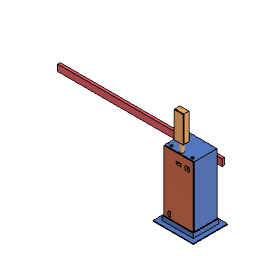
barrier (Autodesk Fusion 360 design; units mm, degrees)
part number: 2026-01-20-15-57-13-019
part number: 2026-01-20-15-58-03-444
part number: 2026-01-20-18-25-53-165
part number: 2026-01-21-16-47-12-671
part number: 2026-01-23-16-32-55-058
Autodesk Fusion 360 part; units mm, degrees
note: some values were not read from the file. Set by a fixed rule: which face or edge a step refers to.
sketch "base" plane through (0, 0, 0) normal (0, 1, 0) x (1, 0, 0) in component "base"
  line L0 (22.5, 0) -> (-22.5, 0)
  line L1 (-22.5, 0) -> (-22.5, -100)
  line L2 (-22.5, -100) -> (22.5, -100)
  line L3 (22.5, -100) -> (22.5, 0)
  line L4 (22.5, 0) -> (-22.5, -100) construction
  line L5 (-22.5, 0) -> (22.5, -100) construction
  point P0 (0, -50)
  dimension "d5" = 45
  dimension "d6" = 100
  constraint horizontal L0
  constraint perpendicular L0 L1
  constraint parallel L0 L2
  constraint parallel L1 L3
  constraint coincident L4 P0
  constraint coincident L5 P0
  constraint midpoint origin L0
  measures "d5" distance of L1.end L2.end
  measures "d6" distance of L0.end L1.end
extrude "Extrude1" add sketch "base" along normal blind 35 makes body 1 in component "base"
shell "Shell1" thickness 1.2 removed faces 1 at (-7.5, 0, 66.6667) on bodies 1 in component "base"
sketch "motor-mount" plane through (0, 33.8, 0) normal (0, -1, 0) x (1, 0, 0) in component "base"
  line L0 (21.3, 1.2) -> (21.3, 98.8)
  line L1 (21.3, 98.8) -> (-21.3, 98.8)
  line L2 (-21.3, 98.8) -> (-21.3, 1.2)
  line L3 (-21.3, 1.2) -> (21.3, 1.2)
  circle A0 centre (0, 85) radius 5
  line L4 (-22.5, 100) -> (22.5, 100)
  line L5 (0, 0) -> (0, 100) construction
  circle A1 centre (17.5, 77) radius 2
  circle A2 centre (-17.5, 77) radius 2
  circle A3 centre (13.2, 45) radius 1
  circle A4 centre (13.2, 15) radius 1
  circle A5 centre (-13.2, 45) radius 1
  circle A6 centre (-13.2, 15) radius 1
  dimension "d15" = 10
  dimension "d16" = 15
  dimension "d17" = 4
  dimension "d18" = 17.5
  dimension "d19" = 8
  dimension "d27" = 2
  dimension "d28" = 13.2
  dimension "d29" = 55
  dimension "d30" = 2
  dimension "d31" = 13.2
  dimension "d32" = 30
  constraint vertical L5.start A0.centre
  constraint coincident L5.start origin
  constraint midpoint L4 L5.end
  constraint symmetric L5 A1 A2
  constraint symmetric L5 A3 A5
  constraint symmetric L5 A4 A6
  measures "d15" diameter of A0
  measures "d16" distance of A0.centre L4
  measures "d17" diameter of A1
  measures "d18" distance of L5 A1.centre
  measures "d19" vertical distance of A0.centre A1.centre
  measures "d27" diameter of A3
  measures "d28" distance of L5 A3.centre
  measures "d29" distance of L4 A3.centre
  measures "d30" diameter of A4
  measures "d31" distance of L5 A4.centre
  measures "d32" distance of A3.centre A4.centre
extrude "Extrude2" cut sketch "motor-mount" against normal through all contours A0 bodies 1 in component "base"
extrude "Extrude3" add sketch "motor-mount" along normal blind 3 contours A1 | A2 bodies 1 in component "base"
extrude "Extrude4" add sketch "motor-mount" along normal blind 4 contours A3 | A4 | A5 | A6 bodies 1 in component "base"
sketch "Sketch1" plane through (0, 35, 0) normal (0, 1, 0) x (-1, 0, 0) in component "arm"
  circle A0 centre (0, 85) radius 5
  line L0 (-22.5, 100) -> (-22.5, 0)
  line L1 (-22.5, 0) -> (22.5, 0)
  line L2 (22.5, 0) -> (22.5, 100)
  line L3 (22.5, 100) -> (-22.5, 100)
  circle A1 centre (0, 85) radius 2.5
  line L4 (2.5, 86.6) -> (-2.5, 86.6)
  line L5 (-2.5, 86.6) -> (-2.5, 83.4)
  line L6 (-2.5, 83.4) -> (2.5, 83.4)
  line L7 (2.5, 83.4) -> (2.5, 86.6)
  line L8 (2.5, 86.6) -> (-2.5, 83.4) construction
  line L9 (-2.5, 86.6) -> (2.5, 83.4) construction
  line L10 (220, 80) -> (-30, 80)
  line L11 (-30, 80) -> (-30, 90)
  line L12 (-30, 90) -> (220, 90)
  line L13 (220, 90) -> (220, 80)
  line L14 (220, 80) -> (-30, 90) construction
  line L15 (-30, 80) -> (220, 90) construction
  point P0 (0, 85)
  point P1 (95, 85)
  dimension "d37" = 5
  dimension "d38" = 15
  dimension "d39" = 5
  dimension "d40" = 3.2
  dimension "d44" = 250
  dimension "d45" = 10
  dimension "d46" = 15
  dimension "d47" = 30
  constraint vertical origin A0.centre
  constraint horizontal L4
  constraint perpendicular L4 L5
  constraint parallel L4 L6
  constraint parallel L5 L7
  constraint coincident L8 P0
  constraint coincident L9 P0
  constraint coincident P0 A0.centre
  constraint horizontal L10
  constraint perpendicular L10 L11
  constraint parallel L10 L12
  constraint parallel L11 L13
  constraint coincident L14 P1
  constraint coincident L15 P1
  measures "d37" diameter of A1
  measures "d38" distance of L3 P0
  measures "d39" distance of L5.end L6.end
  measures "d40" distance of L4.end L5.end
  measures "d44" distance of L11.end L12.end
  measures "d45" distance of L10.end L11.end
  measures "d46" distance of L3 P1
  measures "d47" distance of P0 L11
extrude "Extrude1'" add sketch "Sketch1" along normal blind 4 separate body contours A0 | A0 L2 L10 L12 | A0 L0 L10 L12 | L0 L10 L11 L12 | L2 L10 L12 L13 | A1 L6 L7 | A1 L4 L7 | A1 L4 | A1 L6 | A1 L4 L5 | A1 L5 L6 makes body 2 in component "arm"
sketch "light-box" plane through (0, 0, 0) normal (0, 1, 0) x (1, 0, 0) in component "light-box"
  line L0 (7, -115) -> (-7, -115)
  line L1 (-7, -115) -> (-7, -155)
  line L2 (-7, -155) -> (7, -155)
  line L3 (7, -155) -> (7, -115)
  line L4 (7, -115) -> (-7, -155) construction
  line L5 (-7, -115) -> (7, -155) construction
  line L6 (-22.5, -100) -> (22.5, -100)
  circle A0 centre (0, -148) radius 4.5
  line L7 (7, -139.5) -> (-7, -139.5) construction
  circle A1 centre (0, -131) radius 4.5
  line L8 (7, -138.5) -> (-7, -138.5)
  line L9 (-7, -138.5) -> (-7, -140.5)
  line L10 (-7, -140.5) -> (7, -140.5)
  line L11 (7, -140.5) -> (7, -138.5)
  line L12 (7, -138.5) -> (-7, -140.5) construction
  line L13 (-7, -138.5) -> (7, -140.5) construction
  circle A2 centre (0, -148) radius 5.5
  circle A3 centre (0, -131) radius 5.5
  line L14 (5.7, -116.3) -> (-5.7, -116.3)
  line L15 (-5.7, -116.3) -> (-5.7, -153.7)
  line L16 (-5.7, -153.7) -> (5.7, -153.7)
  line L17 (5.7, -153.7) -> (5.7, -116.3)
  point P0 (0, -135)
  point P1 (0, -85)
  point P2 (0, -139.5)
  dimension "d55" = 14
  dimension "d56" = 40
  dimension "d57" = 15
  dimension "d61" = 9
  dimension "d65" = 7
  dimension "d66" = 8.5
  dimension "d75" = 14
  dimension "d76" = 2
  dimension "d77" = 8.5
  dimension "d78" = 1
  dimension "d79" = 1
  dimension "d146" = -1.3
  constraint horizontal L0
  constraint perpendicular L0 L1
  constraint parallel L0 L2
  constraint parallel L1 L3
  constraint coincident L4 P0
  constraint coincident L5 P0
  constraint vertical origin P0
  constraint vertical A0.centre origin
  constraint coincident L3 L7.start
  constraint coincident L1 L7.end
  constraint perpendicular L1 L7
  constraint symmetric A0 L7 A1
  constraint horizontal L8
  constraint perpendicular L8 L9
  constraint parallel L8 L10
  constraint parallel L9 L11
  constraint coincident L12 P2
  constraint coincident L13 P2
  constraint vertical origin P2
  measures "d55" distance of L1.end L2.end
  measures "d56" distance of L0.end L1.end
  measures "d57" distance of L0 L6
  measures "d61" diameter of A0
  measures "d65" distance of L2 A0.centre
  measures "d66" distance of A0.centre L7
  measures "d75" distance of L9.end L10.end
  measures "d76" distance of L8.end L9.end
  measures "d77" distance of A0.centre P2
extrude "Extrude1''" add sketch "light-box" along normal blind 8 separate body contours L0 L1 L3 L8 L14 L15 L17 | L3 L8 L10 L11 L17 | L1 L8 L9 L10 L15 | L1 L2 L3 L10 L15 L16 L17 | L8 L10 L15 L17 | L8 L14 L15 L17 | L10 L15 L16 L17 | A0 | A1 | A2 | A3 makes body 3 in component "light-box"
shell "Shell1'" thickness 1.2 removed faces 1 at (-2.3333, 0, 122.8333) on bodies 3 in component "light-box"
extrude "Extrude2'" cut sketch "light-box" along normal through all contours A0 | A1 bodies 3 in component "light-box"
sketch "pole" plane through (0, 0, 116.2) normal (0, 0, 1) x (-1, 0, 0) in component "light-box"
  line L0 (5.8, 0) -> (-5.8, 0)
  line L1 (-5.8, 0) -> (-5.8, -6.8)
  line L2 (-5.8, -6.8) -> (5.8, -6.8)
  line L3 (5.8, -6.8) -> (5.8, 0)
  circle A0 centre (0, -4) radius 2
  circle A1 centre (0, -4) radius 2.8
  dimension "d68" = 4
  dimension "d69" = 4
  dimension "d74" = 0.8
  constraint vertical origin A0.centre
  measures "d68" diameter of A0
  measures "d69" distance of origin A0.centre
extrude "Extrude3'" cut sketch "pole" against normal up to surface (1.2 mm away) contours A0 bodies 3 in component "light-box"
extrude "Extrude5" add sketch "light-box" against normal blind 4 from surface at 6.8 contours L3 L8 L10 L11 L17 | L1 L8 L9 L10 L15 | L8 L10 L15 L17 | A2 | A3 bodies 3 in component "light-box"
extrude "Extrude6" add sketch "pole" against normal up to surface (16.2 mm away) separate body contours A1 makes body 4 in component "light-box"
sketch "pole-holes" plane through (0, 0, 100) normal (0, 0, 1) x (-1, 0, 0) in component "base"
  line L0 (22.5, 0) -> (-22.5, 0)
  line L1 (-22.5, 0) -> (-22.5, -35)
  line L2 (-22.5, -35) -> (22.5, -35)
  line L3 (22.5, -35) -> (22.5, 0)
  circle A0 centre (-16, -4) radius 2
  line L4 (0, 0) -> (0, -35) construction
  circle A1 centre (16, -4) radius 2
  dimension "d87" = 4
  dimension "d88" = 4
  dimension "d89" = 16
  constraint coincident L4.start origin
  constraint midpoint L2 L4.end
  constraint symmetric A0 L4 A1
  measures "d87" diameter of A0
  measures "d88" vertical distance of L4.start A0.centre
  measures "d89" horizontal distance of L4.start A0.centre
extrude "Extrude5'" cut sketch "pole-holes" against normal up to surface (1.2 mm away) contours A0 | A1 bodies 1 in component "base"
sketch "door" plane through (0, 0, 0) normal (0, 1, 0) x (1, 0, 0) in component "door"
  line L0 (22.5, 0) -> (-22.5, 0)
  line L1 (-22.5, 0) -> (-22.5, -100)
  line L2 (-22.5, -100) -> (22.5, -100)
  line L3 (22.5, -100) -> (22.5, 0)
  line L4 (22.5, 0) -> (-22.5, -100) construction
  line L5 (-22.5, 0) -> (22.5, -100) construction
  line L6 (21.1, -1.4) -> (-21.1, -1.4)
  line L7 (-21.1, -1.4) -> (-21.1, -98.6)
  line L8 (-21.1, -98.6) -> (21.1, -98.6)
  line L9 (21.1, -98.6) -> (21.1, -1.4)
  line L10 (-19, -27.75) -> (0, -27.75)
  line L11 (0, -27.75) -> (0, -72.25)
  line L12 (0, -72.25) -> (-19, -72.25)
  line L13 (-19, -72.25) -> (-19, -27.75)
  line L14 (-19, -27.75) -> (0, -72.25) construction
  line L15 (0, -27.75) -> (-19, -72.25) construction
  line L16 (-20.2, -26.55) -> (1.2, -26.55)
  line L17 (1.2, -26.55) -> (1.2, -73.45)
  line L18 (1.2, -73.45) -> (-20.2, -73.45)
  line L19 (-20.2, -73.45) -> (-20.2, -26.55)
  line L20 (-20.2, -50) -> (1.2, -50) construction
  line L21 (-9.5, -26.55) -> (-9.5, -73.45) construction
  line L22 (-3.8, -73.45) -> (-3.8, -72.25)
  line L23 (1.2, -68.45) -> (0, -68.45)
  line L24 (-15.2, -73.45) -> (-15.2, -72.25)
  line L25 (-20.2, -68.45) -> (-19, -68.45)
  line L26 (1.2, -31.55) -> (0, -31.55)
  line L27 (-3.8, -26.55) -> (-3.8, -27.75)
  line L28 (-15.2, -26.55) -> (-15.2, -27.75)
  line L29 (-20.2, -31.55) -> (-19, -31.55)
  arc A0 (0, -68.45) -> (-3.8, -72.25) centre (0, -72.25) ccw
  arc A1 (-15.2, -72.25) -> (-19, -68.45) centre (-19, -72.25) ccw
  arc A2 (-3.8, -27.75) -> (0, -31.55) centre (0, -27.75) ccw
  arc A3 (-19, -31.55) -> (-15.2, -27.75) centre (-19, -27.75) ccw
  line L30 (-3.5, -84.6) -> (3.5, -84.6)
  line L31 (3.5, -84.6) -> (3.5, -88.6)
  line L32 (3.5, -88.6) -> (-3.5, -88.6)
  line L33 (-3.5, -88.6) -> (-3.5, -84.6)
  line L34 (-3.5, -84.6) -> (3.5, -88.6) construction
  line L35 (3.5, -84.6) -> (-3.5, -88.6) construction
  circle A4 centre (7.45, -86.6) radius 1
  line L36 (0, -84.6) -> (0, -88.6) construction
  line L37 (0, 0) -> (0, -100) construction
  circle A5 centre (-7.45, -86.6) radius 1
  line L38 (-16.1, -10) -> (-12.1, -10)
  line L39 (-12.1, -10) -> (-12.1, -17)
  line L40 (-12.1, -17) -> (-16.1, -17)
  line L41 (-16.1, -17) -> (-16.1, -10)
  line L42 (-16.1, -10) -> (-12.1, -17) construction
  line L43 (-12.1, -10) -> (-16.1, -17) construction
  line L44 (-16.1, -13.5) -> (-12.1, -13.5) construction
  circle A6 centre (-14.1, -20.95) radius 1
  circle A7 centre (-14.1, -6.05) radius 1
  line L45 (10, -83.55) -> (16.1, -83.55)
  line L46 (16.1, -83.55) -> (16.1, -89.65)
  line L47 (16.1, -89.65) -> (10, -89.65)
  line L48 (10, -89.65) -> (10, -83.55)
  line L49 (10, -83.55) -> (16.1, -89.65) construction
  line L50 (16.1, -83.55) -> (10, -89.65) construction
  point P0 (0, -50)
  point P1 (-9.5, -50)
  point P2 (0, -86.6)
  point P3 (-14.1, -13.5)
  point P4 (13.05, -86.6)
  dimension "d92" = 45
  dimension "d93" = 100
  dimension "d94" = -1.4
  dimension "d99" = 19
  dimension "d100" = 44.5
  dimension "d101" = -1.2
  dimension "d102" = 5
  dimension "d103" = 5
  dimension "d111" = 7
  dimension "d112" = 4
  dimension "d115" = 10
  dimension "d120" = 2
  dimension "d121" = 7.45
  dimension "d125" = 4
  dimension "d126" = 7
  dimension "d127" = 10
  dimension "d128" = 5
  dimension "d132" = 2
  dimension "d134" = 7.45
  dimension "d137" = 6.1
  dimension "d138" = 6.1
  dimension "d140" = 5
  constraint horizontal L0
  constraint perpendicular L0 L1
  constraint parallel L0 L2
  constraint parallel L1 L3
  constraint coincident L4 P0
  constraint coincident L5 P0
  constraint midpoint L0 L37.start
  constraint horizontal L10
  constraint perpendicular L10 L11
  constraint parallel L10 L12
  constraint parallel L11 L13
  constraint coincident L14 P1
  constraint coincident L15 P1
  constraint midpoint P0 L11
  constraint midpoint L19 L20.start
  constraint midpoint L17 L20.end
  constraint midpoint L16 L21.start
  constraint midpoint L18 L21.end
  constraint coincident L18 L22.start
  constraint coincident L12 L22.end
  constraint perpendicular L12 L22
  constraint coincident L17 L23.start
  constraint coincident L11 L23.end
  constraint perpendicular L11 L23
  constraint symmetric L21 L22.start L24.start
  constraint symmetric L21 L22.end L24.end
  constraint symmetric L21 L23.start L25.start
  constraint symmetric L21 L23.end L25.end
  constraint symmetric L20 L22.start L27.start
  constraint symmetric L20 L22.end L27.end
  constraint symmetric L20 L23.start L26.start
  constraint symmetric L20 L23.end L26.end
  constraint symmetric L20 L24.start L28.start
  constraint symmetric L20 L24.end L28.end
  constraint symmetric L20 L25.start L29.start
  constraint symmetric L20 L25.end L29.end
  constraint symmetric L21 A0 A1
  constraint symmetric L20 A0 A2
  constraint symmetric L20 A1 A3
  constraint horizontal L30
  constraint perpendicular L30 L31
  constraint parallel L30 L32
  constraint parallel L31 L33
  constraint coincident L34 P2
  constraint coincident L35 P2
  constraint vertical L37.start P2
  constraint horizontal P2 A4.centre
  constraint midpoint L30 L36.start
  constraint midpoint L32 L36.end
  constraint symmetric A4 L37 A5
  constraint horizontal L38
  constraint perpendicular L38 L39
  constraint parallel L38 L40
  constraint parallel L39 L41
  constraint coincident L42 P3
  constraint coincident L43 P3
  constraint midpoint L41 L44.start
  constraint midpoint L39 L44.end
  constraint vertical P3 A6.centre
  constraint symmetric L44 A6 A7
  constraint horizontal L45
  constraint perpendicular L45 L46
  constraint parallel L45 L47
  constraint parallel L46 L48
  constraint coincident L49 P4
  constraint coincident L50 P4
  constraint horizontal P2 P4
  measures "d92" distance of L1.end L2.end
  measures "d93" distance of L0.end L1.end
  measures "d99" distance of L11.end L12.end
  measures "d100" distance of L10.end L11.end
  measures "d102" distance of L18 L23
  measures "d103" distance of L17 L22
  measures "d111" distance of L31.end L32.end
  measures "d112" distance of L30.end L31.end
  measures "d115" distance of L8 L32
  measures "d120" diameter of A4
  measures "d121" distance of P2 A4.centre
  measures "d125" distance of L39.end L40.end
  measures "d126" distance of L38.end L39.end
  measures "d127" distance of L0 L38
  measures "d128" distance of L7 L41
  measures "d132" diameter of A6
  measures "d134" distance of P3 A6.centre
  measures "d137" distance of L46.end L47.end
  measures "d138" distance of L45.end L46.end
  measures "d140" distance of L9 L46
extrude "Extrude1'''" add sketch "door" against normal blind 1.2 separate body contours L0 L1 L2 L3 | L6 L7 L8 L9 | L10 L13 L16 L19 L28 L29 | L10 L13 A3 | L10 L16 L27 L28 | L10 L11 L12 L13 A0 A1 A2 A3 | L13 L19 L25 L29 | L10 L11 L16 L17 L26 L27 | L10 L11 A2 | L12 L13 A1 | L12 L13 L18 L19 L24 L25 | L11 L17 L23 L26 | L12 L18 L22 L24 | L11 L12 L17 L18 L22 L23 | L11 L12 A0 | L30 L31 L32 L33 | A4 | A5 | L38 L39 L40 L41 | A6 | A7 | L45 L46 L47 L48 makes body 5 in component "door"
extrude "Extrude2''" add sketch "door" along normal blind 2 contours L6 L7 L8 L9 | L10 L13 L16 L19 L28 L29 | L10 L13 A3 | L10 L16 L27 L28 | L10 L11 L12 L13 A0 A1 A2 A3 | L13 L19 L25 L29 | L10 L11 L16 L17 L26 L27 | L10 L11 A2 | L12 L13 A1 | L12 L13 L18 L19 L24 L25 | L11 L17 L23 L26 | L12 L18 L22 L24 | L11 L12 L17 L18 L22 L23 | L11 L12 A0 | L30 L31 L32 L33 | A4 | A5 | L38 L39 L40 L41 | A6 | A7 | L45 L46 L47 L48 bodies 5 in component "door"
extrude "Extrude3''" add sketch "door" along normal blind 4 contours L10 L13 L16 L19 L28 L29 | L10 L13 A3 | L10 L11 L16 L17 L26 L27 | L10 L11 A2 | L12 L13 A1 | L12 L13 L18 L19 L24 L25 | L11 L12 L17 L18 L22 L23 | L11 L12 A0 bodies 5 in component "door"
extrude "Extrude4'" add sketch "door" along normal blind 1.5 from surface at 4 contours L10 L13 L16 L19 L28 L29 | L10 L11 L16 L17 L26 L27 | L12 L13 L18 L19 L24 L25 | L11 L12 L17 L18 L22 L23 bodies 5 in component "door"
extrude "Extrude5''" cut sketch "door" along normal up to surface (2 mm away) contours L30 L31 L32 L33 | L38 L39 L40 L41 | L45 L46 L47 L48 bodies 5 in component "door"
extrude "Extrude6'" cut sketch "door" against normal up to surface (1.2 mm away) contours L30 L31 L32 L33 | L38 L39 L40 L41 | L45 L46 L47 L48 bodies 5 in component "door"
extrude "Extrude7" add sketch "door" along normal blind 4 contours A4 | A5 | A6 | A7 bodies 5 in component "door"
sketch "wiring-hole" plane through (0, 0, 1.2) normal (0, 0, 1) x (-1, 0, 0) in component "base"
  line L0 (21.3, 0) -> (-21.3, 0)
  line L1 (-21.3, 0) -> (-21.3, -33.8)
  line L2 (-21.3, -33.8) -> (21.3, -33.8)
  line L3 (21.3, -33.8) -> (21.3, 0)
  line L4 (-12.5, -10) -> (12.5, -10)
  line L5 (12.5, -10) -> (12.5, -30)
  line L6 (12.5, -30) -> (-12.5, -30)
  line L7 (-12.5, -30) -> (-12.5, -10)
  line L8 (-12.5, -10) -> (12.5, -30) construction
  line L9 (12.5, -10) -> (-12.5, -30) construction
  point P0 (0, -20)
  dimension "d142" = 25
  dimension "d143" = 20
  dimension "d144" = 10
  constraint horizontal L4
  constraint perpendicular L4 L5
  constraint parallel L4 L6
  constraint parallel L5 L7
  constraint coincident L8 P0
  constraint coincident L9 P0
  constraint vertical origin P0
  measures "d142" distance of L5.end L6.end
  measures "d143" distance of L4.end L5.end
  measures "d144" distance of L0 L4
extrude "Extrude6''" cut sketch "wiring-hole" against normal through all contours L4 L5 L6 L7 bodies 1 in component "base"
extrude "Extrude7'" add sketch "light-box" against normal blind 1.2 separate body contours L0 L1 L3 L8 L14 L15 L17 | L3 L8 L10 L11 L17 | L1 L8 L9 L10 L15 | L1 L2 L3 L10 L15 L16 L17 | L8 L10 L15 L17 | L8 L14 L15 L17 | L10 L15 L16 L17 | A0 | A1 | A2 | A3 makes body 6 in component "light-box"
extrude "Extrude8" add sketch "light-box" along normal blind 0.6 contours L8 L10 L15 L17 | L8 L14 L15 L17 | L10 L15 L16 L17 | A0 | A1 | A2 | A3 bodies 6 in component "light-box"
sketch "Sketch5" plane through (0, 0, 0) normal (0, 0, 1) x (1, 0, 0) in component "base"
  line L0 (-22.5, 0) -> (-22.5, 35)
  line L1 (-22.5, 35) -> (22.5, 35)
  line L2 (22.5, 0) -> (22.5, 35)
  line L3 (22.5, 0) -> (22.5, -1.2)
  line L4 (22.5, -1.2) -> (-22.5, -1.2)
  line L5 (-22.5, 0) -> (-22.5, -1.2)
  line L6 (22.6, -1.4) -> (-22.6, -1.4)
  line L7 (-22.6, -1.4) -> (-22.6, 35)
  line L8 (-22.6, 35) -> (22.6, 35)
  line L9 (22.6, 35) -> (22.6, -1.4)
  line L10 (22.6, -1.4) -> (-22.6, 35) construction
  line L11 (-22.6, -1.4) -> (22.6, 35) construction
  line L12 (23.8, 36.2) -> (23.8, -2.6)
  line L13 (23.8, -2.6) -> (-23.8, -2.6)
  line L14 (-23.8, -2.6) -> (-23.8, 36.2)
  line L15 (-23.8, 36.2) -> (23.8, 36.2)
  line L16 (30.6, -9.4) -> (-30.6, -9.4)
  line L17 (-30.6, -9.4) -> (-30.6, 43)
  line L18 (-30.6, 43) -> (30.6, 43)
  line L19 (30.6, 43) -> (30.6, -9.4)
  point P0 (0, 16.8)
  dimension "d151" = 45.2
  dimension "d152" = 36.4
  constraint horizontal L6
  constraint perpendicular L6 L7
  constraint parallel L6 L8
  constraint parallel L7 L9
  constraint coincident L10 P0
  constraint coincident L11 P0
  constraint midpoint L1 L8
  measures "d151" distance of L7.end L8.end
  measures "d152" distance of L6.end L7.end
extrude "Extrude7''" add sketch "Sketch5" along normal blind 1.2 separate body contours L0 L2 L3 L4 L5 L6 L7 L8 L9 | L12 L13 L14 L15 | L16 L17 L18 L19 makes body 7 in component "base"
extrude "Extrude8'" add sketch "Sketch5" along normal blind 8 contours L12 L13 L14 L15 bodies 7 in component "base"
component "base" placed x (1, 0, 0) y (0, 1, 0) z (0, 0, 1) at (0, 0, 0)
component "arm" placed x (1, 0, 0) y (0, 1, 0) z (0, 0, 1) at (0, 0, 0)
component "light-box" placed x (1, 0, 0) y (0, 1, 0) z (0, 0, 1) at (0, 0, 0)
component "door" placed x (1, 0, 0) y (0, 1, 0) z (0, 0, 1) at (0, 0, 0) in component "base"
equation "base_x = 45 mm"
equation "base_z = 100 mm"
equation "base_y = 35 mm"
equation "base_wall_thickness = 1.2 mm"
equation "d5 = base_x"
equation "d6 = base_z"
equation "d7 = base_y"
equation "d9 = base_wall_thickness"
equation "motor_hole_diameter = 10 mm"
equation "motor_mount_diameter = 4 mm"
equation "motor_mount_offset_x = 17.5 mm"
equation "motor_mount_hole_offset_z = 8 mm"
equation "motor_hole_offset_z = 15 mm"
equation "d15 = motor_hole_diameter"
equation "d16 = motor_hole_offset_z"
equation "d17 = motor_mount_diameter"
equation "d18 = motor_mount_offset_x"
equation "d19 = motor_mount_hole_offset_z"
equation "motor_control_board_hole_diameter = 2 mm"
equation "motor_control_board_hole_offset_x = 13.2 mm"
equation "motor_control_board_hole_offset_z = 55 mm"
equation "motor_control_board_hole_spacing_z = 30 mm"
equation "d27 = motor_control_board_hole_diameter"
equation "d28 = motor_control_board_hole_offset_x"
equation "d29 = motor_control_board_hole_offset_z"
equation "d30 = motor_control_board_hole_diameter"
equation "d31 = motor_control_board_hole_offset_x"
equation "d32 = motor_control_board_hole_spacing_z"
equation "motor_spindle_diameter = 5 mm"
equation "motor_spindle_flat = 3.2 mm"
equation "d37 = motor_spindle_diameter"
equation "d38 = motor_hole_offset_z"
equation "d39 = motor_spindle_diameter"
equation "d40 = motor_spindle_flat"
equation "arm_x = 250 mm"
equation "arm_z = 10 mm"
equation "arm_y = 4 mm"
equation "d44 = arm_x"
equation "d45 = arm_z"
equation "d46 = motor_hole_offset_z"
equation "d47 = arm_offset_x"
equation "arm_offset_x = 30 mm"
equation "d49 = arm_y"
equation "light_box_x = 14 mm"
equation "light_box_z = 40 mm"
equation "light_box_y = 8 mm"
equation "light_box_pole_diameter = 4 mm"
equation "d55 = light_box_x"
equation "d56 = light_box_z"
equation "d58 = light_box_y"
equation "d60 = base_wall_thickness"
equation "light_box_bulb_diameter = 9 mm"
equation "light_box_bulb_spacing = 17 mm"
equation "light_box_bulb_offset_z = 7 mm"
equation "d65 = light_box_bulb_offset_z"
equation "d66 = light_box_bulb_spacing / 2"
equation "d68 = light_box_pole_diameter"
equation "d69 = light_box_y / 2"
equation "d75 = light_box_x"
equation "d77 = light_box_bulb_spacing / 2"
equation "d78 = light_box_bulb_shade_thickness"
equation "d79 = light_box_bulb_shade_thickness"
equation "light_box_bleed_stop_height = 2 mm"
equation "light_box_bulb_shade_thickness = 1 mm"
equation "d87 = light_box_pole_diameter"
equation "d88 = light_box_pole_diameter"
equation "d89 = ( light_box_z / 2 ) - light_box_pole_diameter"
equation "d92 = base_x"
equation "d93 = base_z"
equation "d94 = -base_wall_thickness - 0.2 mm"
equation "d95 = -base_wall_thickness"
equation "d102 = mcu_standoff_length"
equation "d103 = mcu_standoff_length"
equation "mcu_standoff_thickness = 1.2 mm"
equation "mcu_standoff_length = 5 mm"
equation "d111 = switch_hole_y"
equation "d112 = switch_hole_z"
equation "switch_hole_y = 7 mm"
equation "switch_hole_z = 4 mm"
equation "d115 = toggle_switch_offset_z"
equation "d120 = switch_mount_diameter"
equation "d121 = switch_mount_offset"
equation "switch_mount_diameter = 2 mm"
equation "d125 = switch_hole_z"
equation "d126 = switch_hole_y"
equation "d127 = power_switch_offset_z"
equation "d128 = power_switch_offset_y"
equation "power_switch_offset_y = 5 mm"
equation "power_switch_offset_z = 10 mm"
equation "toggle_switch_offset_z = 10 mm"
equation "d132 = switch_mount_diameter"
equation "switch_mount_offset = 7.45 mm"
equation "d134 = switch_mount_offset"
equation "jog_button_y = 6.1 mm"
equation "jog_button_z = 6.1 mm"
equation "d137 = jog_button_y"
equation "d138 = jog_button_z"
equation "d140 = jog_button_offset_x"
equation "jog_button_offset_x = 5 mm"
equation "d146 = -base_wall_thickness - 0.1 mm"
equation "d147 = -base_wall_thickness"
equation "d151 = base_x + ( clearance_tolerance * 2 )"
equation "d152 = base_y + base_wall_thickness + ( clearance_tolerance * 2 )"
equation "clearance_tolerance = 0.1 mm"
equation "d154 = -base_wall_thickness"
equation "d155 = -base_fixing_offset"
equation "base_fixing_offset = 8 mm"
named bodies: "cabinet", "arm", "light-box", "pole", "door", "light-box-back", "floor fixing"
